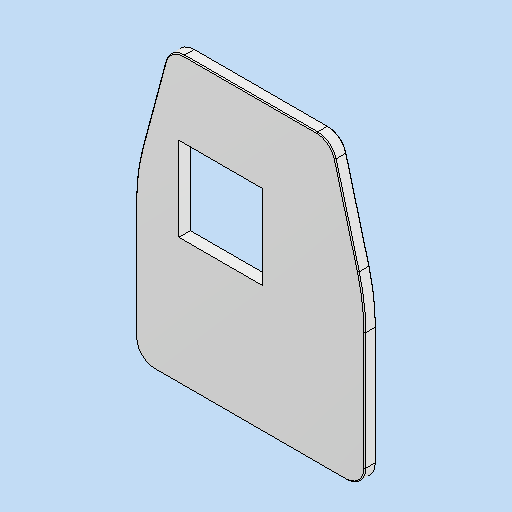
# Autodesk Inventor part: tc-front-panel
Saved by Autodesk Inventor 2025 (Build 290162000, 162)
## iProperties
Created: 2025-06-05
Part Number: tc-front-panel
Material: ABS Plastic
Document SubType Name: Modeling
Designer: queezz
Density: 1.06 g/cm^3
Appearance: Smooth - White
Author: queezz
Autodesk Inventor part; units mm, degrees
ref_plane "YZ Plane" through (0, 0, 0) normal (1, 0, 0) x (0, 1, 0)
ref_plane "XZ Plane" through (0, 0, 0) normal (0, 1, 0) x (-1, 0, 0)
ref_plane "XY Plane" through (0, 0, 0) normal (0, 0, 1) x (1, 0, 0)
sketch "Sketch1" plane through (0, 0, 0) normal (0, 0, 1) x (1, 0, 0)
  line L0 (-60, 75) -> (60, 75)
  line L1 (60, 75) -> (60, -75)
  line L2 (60, -75) -> (-60, -75)
  line L3 (-60, -75) -> (-60, 75)
  point P0 (0, 0)
  point P1 (60, 0)
  point P2 (0, 75)
  dimension "d0" = 120
  dimension "d1" = 150
  constraints: 8 end point, 2 midpoint, 2 parallel, 1 horizontal, 1 horizontal alignment, 1 perpendicular, 1 vertical alignment
  measures "d0" distance of L0.start L0.end
  measures "d1" distance of L0.end L1.end
extrude "Extrusion1" add sketch "Sketch1" along normal blind 6
sketch "Sketch2" plane through (0, 0, 6) normal (0, 0, 1) x (1, 0, 0)
  line L0 (-37.3514, 35.3082) -> (6.6486, 35.3082)
  line L1 (6.6486, 35.3082) -> (6.6486, -8.6918)
  line L2 (6.6486, -8.6918) -> (-37.3514, -8.6918)
  line L3 (-37.3514, -8.6918) -> (-37.3514, 35.3082)
  point P0 (0, 0)
  dimension "d4" = 44
  dimension "d5" = 44
  constraints: 8 end point, 2 parallel, 1 horizontal, 1 perpendicular
  measures "d4" distance of L0.start L0.end
  measures "d5" distance of L0.end L1.end
extrude "Hole" cut sketch "Sketch2" against normal through all
sketch "Sketch3" plane through (0, 0, 6) normal (0, 0, 1) x (1, 0, 0)
  line L0 (6.6486, 35.3082) -> (6.6486, -8.6918) projected
  line L1 (6.6486, -8.6918) -> (-37.3514, -8.6918) projected
  line L2 (-37.3514, -8.6918) -> (-37.3514, 35.3082) projected
  line L3 (-37.3514, 35.3082) -> (6.6486, 35.3082) projected
  line L4 (-60, -75) -> (60, -75) projected
  line L5 (60, -75) -> (60, 75) projected
  line L6 (60, 75) -> (-60, 75) projected
  line L7 (-60, 75) -> (-60, -75) projected
  line L8 (-60, 9.6891) -> (-42.5, 75)
  line L9 (42.5, 75) -> (60, 9.6891)
  line L10 (-42.5, 75) -> (42.5, 75)
  line L11 (60, 75) -> (-60, 75) construction
  point P0 (0, 0)
  point P1 (0, 75)
  dimension "d9" = 15
  dimension "d10" = 85
  constraints: 6 end point, 4 point on line, 1 collinear, 1 equal length, 1 horizontal alignment, 1 midpoint, 1 vertical alignment
  measures "d9" angle of L5 L9
  measures "d10" distance of L9.start L8.end
extrude "Extrusion3" cut sketch "Sketch3" against normal through all contours L7 L6 L8 | L9 L6 L5
fillet "Fillet1" radius 10 4 edges at (60, -75, 3) (-60, -75, 3) (-42.5, 75, 3) (42.5, 75, 3)
fillet "Fillet2" radius 100 2 edges at (60, 9.6891, 3) (-60, 9.6891, 3)
chamfer "Chamfer1" distance 0.5 angle 45 24 edges at (0, 75, 6) (-40.9143, 72.9335, 6) (-50.5393, 44.997, 6) (-59.1445, 9.5765, 6) (-60, -34.2381, 6) (-57.0711, -72.0711, 6) (0, -75, 6) (57.0711, -72.0711, 6) (60, -34.2381, 6) (59.1445, 9.5765, 6) (50.5393, 44.997, 6) (40.9143, 72.9335, 6) (0, 75, 0) (-40.9143, 72.9335, 0) (-50.5393, 44.997, 0) (-59.1445, 9.5765, 0) (-60, -34.2381, 0) (-57.0711, -72.0711, 0) (0, -75, 0) (57.0711, -72.0711, 0) (60, -34.2381, 0) (59.1445, 9.5765, 0) (50.5393, 44.997, 0) (40.9143, 72.9335, 0)
equation "\"d0\" = width"
equation "\"d1\" = hight"
equation "\"hight\" = 150"
equation "\"width\" = 120"
body "Solid1"
